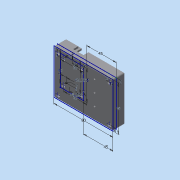
# Autodesk Inventor part: Base_V2
Saved by Autodesk Inventor 2015 (Build 190159000, 159)
## iProperties
Created: 2014-12-24
Part Number: Base_V2
Material: Generic
Document SubType Name: Modeling
Designer: Openlab
Density: 1 g/cm^3
Appearance: Default
Mass: 62.6091 g
Surface Area: 292.318 cm^2
Volume: 62.6091 cm^3
Author: Openlab
Autodesk Inventor part; units mm, degrees
ref_plane "YZ Plane" through (0, 0, 0) normal (1, 0, 0) x (0, 1, 0)
ref_plane "XZ Plane" through (0, 0, 0) normal (0, 1, 0) x (-1, 0, 0)
sketch "Sketch1" plane through (0, 0, 0) normal (0, 1, 0) x (-1, 0, 0)
  line L0 (90, 0) -> (0, 0)
  line L1 (0, 0) -> (0, -68)
  line L2 (0, -68) -> (90, -68)
  line L3 (90, -68) -> (90, 0)
  line L4 (85, -5) -> (67.5, -5)
  line L5 (5, -5) -> (5, -63)
  line L6 (5, -63) -> (85, -63)
  line L7 (85, -63) -> (85, -5)
  line L8 (35, -6.5) -> (22, -6.5)
  line L9 (22, -6.5) -> (22, -19.5)
  line L10 (22, -19.5) -> (35, -19.5)
  line L11 (35, -42.5) -> (22, -42.5)
  line L12 (22, -42.5) -> (22, -55.5)
  line L13 (22, -55.5) -> (35, -55.5)
  line L14 (85, -5) -> (81, -5)
  line L15 (81, -5) -> (81, -9)
  line L16 (81, -9) -> (85, -9)
  line L17 (85, -9) -> (85, -5)
  line L18 (85, -63) -> (81, -63)
  line L19 (81, -63) -> (81, -59)
  line L20 (81, -59) -> (85, -59)
  line L21 (85, -59) -> (85, -63)
  line L22 (5, -5) -> (9, -5)
  line L23 (9, -5) -> (9, -9)
  line L24 (9, -9) -> (5, -9)
  line L25 (5, -9) -> (5, -5)
  line L26 (5, -63) -> (9, -63)
  line L27 (9, -63) -> (9, -59)
  line L28 (9, -59) -> (5, -59)
  line L29 (5, -59) -> (5, -63)
  line L30 (67.5, -5) -> (67.5, -2.6)
  line L31 (67.5, -2.6) -> (57.5, -2.6)
  line L32 (57.5, -2.6) -> (57.5, -5)
  line L33 (67.5, -5) -> (72.2264, -5) construction
  line L34 (85, -5) -> (67.5, -5)
  line L35 (72.2264, -5) -> (57.5, -5) construction
  line L36 (57.5, -5) -> (55.2, -5)
  line L37 (12, -59) -> (12, -5)
  line L38 (40, -59) -> (12, -59)
  line L39 (12, -5) -> (5, -5)
  line L40 (36.85, -54) -> (38.15, -54)
  line L41 (38.15, -44) -> (36.85, -44)
  line L42 (35, -50.5) -> (36.85, -50.5)
  line L43 (38.15, -50.5) -> (40, -50.5)
  line L44 (40, -47.5) -> (38.15, -47.5)
  line L45 (36.85, -47.5) -> (35, -47.5)
  line L46 (36.85, -36) -> (38.15, -36)
  line L47 (38.15, -26) -> (36.85, -26)
  line L48 (40, -32.5) -> (38.15, -32.5)
  line L49 (36.85, -32.5) -> (35, -32.5)
  line L50 (40, -29.5) -> (38.15, -29.5)
  line L51 (36.85, -29.5) -> (35, -29.5)
  line L52 (35.95, -18) -> (39.05, -18)
  line L53 (39.05, -8) -> (35.95, -8)
  line L54 (35, -14.5) -> (35.95, -14.5)
  line L55 (39.05, -14.5) -> (40, -14.5)
  line L56 (35, -11.5) -> (35.95, -11.5)
  line L57 (39.05, -11.5) -> (40, -11.5)
  line L58 (12, -51.5) -> (22, -51.5)
  line L59 (12, -46.5) -> (22, -46.5)
  line L60 (12, -33.5) -> (22, -33.5)
  line L61 (12, -28.5) -> (22, -28.5)
  line L62 (12, -15.5) -> (22, -15.5)
  line L63 (12, -10.5) -> (22, -10.5)
  line L64 (42, -5) -> (42, -55)
  line L65 (57.5, -5) -> (44, -5)
  line L66 (42, -5) -> (40, -5)
  line L67 (42, -5) -> (44, -5)
  line L68 (10, -5) -> (10, -63)
  line L69 (9, -59) -> (9, -5)
  line L70 (2.6, -65.4) -> (2.6, -2.6)
  line L71 (2.6, -2.6) -> (87.4, -2.6)
  line L72 (87.4, -2.6) -> (87.4, -65.4)
  line L73 (87.4, -65.4) -> (2.6, -65.4)
  line L74 (42, -55) -> (44, -55)
  line L75 (44, -55) -> (44, -5)
  line L76 (42.1668, -13) -> (13.95, -13) construction
  line L77 (35, -6.5) -> (35, -19.5)
  line L78 (37.5, -5.5957) -> (37.5, -61.9523) construction
  line L79 (39.05, -8) -> (39.05, -18)
  line L80 (35.95, -8) -> (35.95, -18)
  line L81 (44.1467, -31) -> (11.3232, -31) construction
  line L82 (38.15, -26) -> (38.15, -36)
  line L83 (36.85, -26) -> (36.85, -36)
  line L84 (13.6727, -49) -> (43.8542, -49) construction
  line L85 (38.15, -44) -> (38.15, -54)
  line L86 (36.85, -44) -> (36.85, -54)
  line L87 (40, -5) -> (40, -59)
  line L88 (35, -42.5) -> (35, -55.5)
  line L89 (35, -24.5) -> (22, -24.5)
  line L90 (22, -24.5) -> (22, -37.5)
  line L91 (22, -37.5) -> (35, -37.5)
  line L92 (35, -37.5) -> (35, -24.5)
  line L93 (44, -63) -> (44, -61)
  line L94 (44, -61) -> (38, -61)
  line L95 (38, -61) -> (38, -63)
  line L96 (28.5, -5.8794) -> (28.5, -56.7788) construction
  point P0 (28.5, -13)
  point P1 (28.5, -31)
  point P2 (28.5, -49)
  dimension "d1" = 5
  dimension "d2" = 5
  dimension "d3" = 5
  dimension "d4" = 5
  dimension "d32" = 13
  dimension "d55" = 4
  dimension "d56" = 4
  dimension "d57" = 4
  dimension "d58" = 4
  dimension "d60" = 4
  dimension "d61" = 4
  dimension "d62" = 4
  dimension "d186" = 10
  dimension "d197" = 68
  dimension "d234" = 1.3
  dimension "d235" = 10
  dimension "d253" = 3
  dimension "d254" = 1.3
  dimension "d255" = 10
  dimension "d265" = 3
  dimension "d266" = 3.1
  dimension "d267" = 10
  dimension "d273" = 5
  dimension "d275" = 5
  dimension "d277" = 5
  dimension "d297" = 10
  dimension "d364" = 22.5
  dimension "d371" = 2.6
  dimension "d372" = 2.6
  dimension "d373" = 2.6
  dimension "d374" = 2.6
  dimension "d386" = 2
  dimension "d395" = 13
  dimension "d401" = 18
  dimension "d402" = 18
  dimension "d405" = 13
  dimension "d406" = 5
  dimension "d407" = 2
  dimension "d408" = 3
  dimension "d410" = 13
  dimension "d441" = 2
  dimension "d444" = 13
  dimension "d449" = 5
  dimension "d451" = 6.5
  dimension "d452" = 12.5
  dimension "d453" = 3.5
  dimension "d454" = 1
  dimension "d455" = 2
  dimension "d456" = 6
  dimension "d461" = 4
  dimension "d462" = 90
  dimension "d471" = 50
  constraints: 194 end point, 48 point on line, 32 perpendicular, 30 parallel, 25 horizontal, 13 collinear, 11 vertical, 1 coincident, 17 other
  measures "d1" distance between parallel lines of L2 L6
  measures "d2" distance between parallel lines of L7 L3
  measures "d3" distance between parallel lines of L1 L5
  measures "d4" distance between parallel lines of L4 L0
  measures "d32" distance of L13.end L11.start
  measures "d55" distance of L16.end L15.end
  measures "d56" distance of L15.end L14.end
  measures "d57" distance of L19.end L20.end
  measures "d58" distance of L18.end L19.end
  measures "d60" distance of L22.end L23.end
  measures "d61" distance of L28.end L27.end
  measures "d62" distance of L27.end L26.end
  measures "d186" distance of L30.end L31.end
  measures "d197" distance between parallel lines of L0 L2
  measures "d234" distance of L41.start L41.end
  measures "d235" distance of L40.end L41.start
  measures "d253" distance between parallel lines of L45 L42
  measures "d254" distance of L47.end L47.start
  measures "d255" distance of L47.start L46.end
  measures "d265" distance between parallel lines of L50 L48
  measures "d266" distance of L53.end L53.start
  measures "d267" distance of L53.start L52.end
  measures "d273" distance between parallel lines of L63 L62
  measures "d275" distance between parallel lines of L61 L60
  measures "d277" distance between parallel lines of L58 L59
  measures "d297" distance between parallel lines of L12 L37
  measures "d364" distance between parallel lines of L3 L30
  measures "d371" distance between parallel lines of L1 L70
  measures "d372" distance between parallel lines of L0 L71
  measures "d373" distance between parallel lines of L2 L73
  measures "d374" distance between parallel lines of L3 L72
  measures "d386" distance of L64.end L74.end
  measures "d395" distance between parallel lines of L10 L8
  measures "d401" distance between parallel lines of L81 L76
  measures "d402" distance between parallel lines of L84 L81
  measures "d405" distance between parallel lines of L12 L88
  measures "d406" distance between parallel lines of L88 L87
  measures "d407" distance between parallel lines of L87 L64
  measures "d408" distance between parallel lines of L54 L56
  measures "d410" distance between parallel lines of L91 L89
  measures "d441" distance between parallel lines of L68 L37
  measures "d444" distance between parallel lines of L0 L76
  measures "d449" distance between parallel lines of L0 L22
  measures "d451" distance between parallel lines of L0 L8
  measures "d452" distance between parallel lines of L2 L13
  measures "d453" distance between parallel lines of L38 L13
  measures "d454" distance between parallel lines of L27 L68
  measures "d455" distance of L93.start L93.end
  measures "d456" distance of L93.end L94.end
  measures "d461" distance of L23.end L24.end
  measures "d462" distance between parallel lines of L1 L3
  measures "d471" distance between parallel lines of L74 L65
extrude "Extrusion1" add sketch "Sketch1" against normal blind 5 contours L3 L2 L1 L0 | L7 L16 L15 L4 | L4 L30 L71 L72 L73 L70 L32 L36 L65 L67 L66 L87 L57 L79 L53 L80 L56 L77 L8 L9 L63 L37 L39 L22 L5 L6 L7 | L15 L16 L7 L20 L19 L6 L93 L94 L95 L68 L39 L37 L38 L87 L66 L64 L74 L75 L65 L36 L32 L31 L30 L4 | L7 L6 L19 L20 | L6 L95 L94 L93 | L75 L74 L64 L67 | L6 L27 L69 L23 L39 L68 | L6 L5 L28 L27 | L28 L5 L24 L69 | L23 L24 L5 L22 | L87 L55 L79 L57 | L63 L9 L62 L37 | L79 L52 L80 L53 | L87 L50 L82 L47 L83 L51 L92 L89 L90 L61 L37 L62 L9 L10 L77 L54 L80 L52 L79 L55 | L9 L8 L77 L10 | L87 L48 L82 L50 | L61 L90 L60 L37 | L82 L46 L83 L47 | L87 L44 L85 L41 L86 L45 L88 L11 L12 L59 L37 L60 L90 L91 L92 L49 L83 L46 L82 L48 | L90 L89 L92 L91 | L80 L54 L77 L56 | L87 L43 L85 L44 | L59 L12 L58 L37 | L85 L40 L86 L41 | L87 L38 L37 L58 L12 L13 L88 L42 L86 L40 L85 L43 | L12 L11 L88 L13 | L83 L49 L92 L51 | L86 L42 L88 L45
sketch "Sketch3" plane through (0, 0, 0) normal (0, 1, 0) x (-1, 0, 0)
  line L0 (45, -5) -> (45, -50)
  line L1 (80, -50) -> (80, -5)
  line L2 (80, -5) -> (45, -5)
  line L3 (45, -50) -> (80, -50)
  line L4 (71.771, -5) -> (53.229, -5)
  line L5 (53.229, -5) -> (53.229, -48.18)
  line L6 (53.229, -48.18) -> (71.771, -48.18)
  line L7 (71.771, -48.18) -> (71.771, -5)
  line L8 (62.5, 1.7089) -> (62.5, -57.768) construction
  line L9 (66.5, -10) -> (58.5, -10)
  line L10 (58.5, -10) -> (58.5, -5)
  line L11 (58.5, -5) -> (66.5, -5)
  line L12 (66.5, -5) -> (66.5, -10)
  circle A0 centre (76, -45) radius 3.5
  circle A1 centre (49, -45) radius 3.5
  circle A2 centre (76, -10) radius 3.5
  circle A3 centre (49, -10) radius 3.5
  point P0 (0, 0)
  dimension "d37" = 35
  dimension "d38" = 45
  dimension "d39" = 5
  dimension "d40" = 4
  dimension "d41" = 5
  dimension "d42" = 4
  dimension "d43" = 18.542
  dimension "d44" = 43.18
  dimension "d45" = 8
  dimension "d46" = 5
  dimension "d47" = 45
  dimension "d48" = 5
  dimension "d148" = 7
  dimension "d149" = 7
  dimension "d150" = 7
  dimension "d151" = 7
  constraints: 26 end point, 6 parallel, 5 coincident, 4 centre point, 4 horizontal alignment, 3 horizontal, 3 perpendicular, 2 vertical alignment, 1 vertical, 3 other
  measures "d37" distance of L1.start L0.end
  measures "d38" distance of L1.end L1.start
  measures "d39" distance from line of L2 point (76, -10)
  measures "d40" distance from line of L1 point (76, -45)
  measures "d41" distance from line of L3 point (76, -45)
  measures "d42" distance from line of L0 point (49, -10)
  measures "d43" distance of L5.end L6.end
  measures "d44" distance of L4.end L5.end
  measures "d45" distance of L9.start L9.end
  measures "d46" distance of L11.end L9.start
  measures "d47" distance from line of point (0, 0) L0
  measures "d48" vertical distance of point (0, 0) point (45, -5)
  measures "d148" diameter of A0
  measures "d149" diameter of A1
  measures "d150" diameter of A2
  measures "d151" diameter of A3
extrude "Extrusion4" add sketch "Sketch3" along normal blind 2 contours A0 | A1 | A2 | A3
sketch "Sketch5" plane through (0, -5, 0) normal (0, -1, 0) x (1, 0, 0)
  line L0 (-90, 0) -> (0, 0)
  line L1 (0, 0) -> (0, -68)
  line L2 (0, -68) -> (-90, -68)
  line L3 (-90, -68) -> (-90, 0)
  line L4 (-45, -5) -> (-45, -50)
  line L5 (-80, -50) -> (-80, -5)
  line L6 (-45, -50) -> (-80, -50)
  line L7 (-80, -5) -> (-45, -5)
  point P0 (-84, -62)
  point P1 (-84, -6)
  point P2 (-6, -6)
  point P3 (-6, -62)
  point P4 (-49, -10)
  point P5 (-76, -10)
  point P6 (-76, -45)
  point P7 (-49, -45)
  dimension "d310" = 90
  dimension "d311" = 68
  dimension "d314" = 6
  dimension "d315" = 6
  dimension "d316" = 6
  dimension "d317" = 6
  dimension "d326" = 45
  dimension "d342" = 35
  dimension "d347" = 4
  dimension "d352" = 4
  dimension "d353" = 5
  dimension "d354" = 5
  dimension "d355" = 45
  dimension "d356" = 5
  constraints: 16 end point, 4 horizontal alignment, 4 parallel, 4 vertical alignment, 2 coincident, 2 perpendicular, 1 horizontal
  measures "d310" distance of L1.end L2.end
  measures "d311" distance of L0.end L1.end
  measures "d314" distance from line of L0 point (-6, -6)
  measures "d315" distance from line of L1 point (-6, -6)
  measures "d316" distance from line of L2 point (-6, -62)
  measures "d317" distance from line of L3 point (-84, -6)
  measures "d326" distance of L4.end L4.start
  measures "d342" distance of L5.end L4.start
  measures "d347" distance from line of L5 point (-76, -10)
  measures "d352" distance from line of L4 point (-49, -10)
  measures "d353" distance from line of L7 point (-49, -10)
  measures "d354" distance from line of L6 point (-49, -45)
  measures "d355" distance between parallel lines of L1 L4
  measures "d356" distance between parallel lines of L0 L7
hole "Hole22" at (-49, -5, -10) at (-76, -5, -10) at (-76, -5, -45) at (-49, -5, -45) direction (0, 1, 0) diameter 4 end through all counterbore diameter 6.5 counterbore depth 3
extrude "Extrusion16" add sketch "Sketch1" along normal blind 12.5
sketch "Sketch7" plane through (-90, -5, 0) normal (0, 0, 1) x (1, 0, 0)
  line L0 (19.5, 17.5) -> (35.5, 17.5)
  line L1 (35.5, 17.5) -> (35.5, 10)
  line L2 (35.5, 10) -> (19.5, 10)
  line L3 (19.5, 10) -> (19.5, 17.5)
  line L4 (0, 17.5) -> (0, 0) projected
  point P0 (90, 5)
  dimension "d380" = 16
  dimension "d381" = 7.5
  dimension "d382" = 19.5
  dimension "d383" = 10
  constraints: 8 end point, 2 parallel, 1 horizontal, 1 perpendicular
  measures "d380" distance of L1.end L2.end
  measures "d381" distance of L0.end L1.end
  measures "d382" distance between parallel lines of L4 L3
  measures "d383" distance from line of L4.end L2
extrude "Extrusion17" cut sketch "Sketch7" against normal blind 12.5
extrude "Extrusion19" add sketch "Sketch1" along normal blind 15 contours L7 L16 L15 L4 | L4 L30 L71 L72 L73 L70 L32 L36 L65 L67 L66 L87 L57 L79 L53 L80 L56 L77 L8 L9 L63 L37 L39 L22 L5 L6 L7 | L7 L6 L19 L20 | L6 L5 L28 L27 | L23 L24 L5 L22 | L87 L50 L82 L47 L83 L51 L92 L89 L90 L61 L37 L62 L9 L10 L77 L54 L80 L52 L79 L55 | L87 L44 L85 L41 L86 L45 L88 L11 L12 L59 L37 L60 L90 L91 L92 L49 L83 L46 L82 L48 | L87 L38 L37 L58 L12 L13 L88 L42 L86 L40 L85 L43
extrude "Extrusion20" add sketch "Sketch1" along normal blind 7.4 contours L87 L55 L79 L57 | L63 L9 L62 L37 | L87 L48 L82 L50 | L61 L90 L60 L37 | L80 L54 L77 L56 | L87 L43 L85 L44 | L59 L12 L58 L37 | L83 L49 L92 L51 | L86 L42 L88 L45
extrude "Extrusion21" add sketch "Sketch1" along normal blind 2.5 contours L79 L52 L80 L53 | L82 L46 L83 L47 | L85 L40 L86 L41
hole "Hole21" at (-6, -5, -6) at (-84, -5, -6) at (-84, -5, -62) at (-6, -5, -62) direction (0, 1, 0) diameter 4 end through all counterbore diameter 6.5 counterbore depth 3
fillet "Fillet4" radius 2.5 6 edges at (-17, 7.4, -51.5) (-17, 7.4, -46.5) (-17, 7.4, -33.5) (-17, 7.4, -28.5) (-17, 7.4, -15.5) (-17, 7.4, -10.5)
sketch "Sketch9" plane through (-12, 0, -5) normal (1, 0, 0) x (0, 0, -1)
  point P0 (-5, 0)
ref_plane "Work Plane1" through (-12, 0, -5) normal (1, 0, 0) x (0, 0, -1)
sketch "Sketch10" plane through (-12, -5, 0) normal (1, 0, 0) x (0, 0, -1)
  line L0 (80, 0) -> (0, 0) construction
  arc A0 (10, 15) -> (16, 15) centre (13, 15) ccw
  arc A1 (28, 15) -> (34, 15) centre (31, 15) ccw
  arc A2 (46, 15) -> (52, 15) centre (49, 15) ccw
  line L1 (10, 15) -> (10, 20)
  line L2 (10, 20) -> (16, 20)
  line L3 (16, 20) -> (16, 15)
  line L4 (28, 15) -> (28, 20)
  line L5 (28, 20) -> (34, 20)
  line L6 (34, 20) -> (34, 15)
  line L7 (46, 15) -> (46, 20)
  line L8 (46, 20) -> (52, 20)
  line L9 (52, 20) -> (52, 15)
  line L10 (59, 5) -> (59, 20) projected
  line L11 (51.5, 20) -> (59, 20) projected
  line L12 (9, 5) -> (59, 5) projected
  line L13 (0, 0) -> (0, 17.5) projected
  point P0 (0, 5)
  point P1 (59, 7.5)
  dimension "d423" = 18
  dimension "d424" = 18
  dimension "d425" = 6
  dimension "d426" = 6
  dimension "d427" = 6
  dimension "d443" = 10
  dimension "d460" = 13
  constraints: 18 end point, 6 point on circle, 6 tangent, 5 perpendicular, 3 centre point, 3 coincident, 2 collinear, 2 horizontal alignment, 2 point on line, 2 vertical, 1 parallel
  measures "d423" distance of point (31, 15) point (13, 15)
  measures "d424" distance of point (49, 15) point (31, 15)
  measures "d425" diameter of A0
  measures "d426" diameter of A1
  measures "d427" diameter of A2
  measures "d443" distance from line of L12 A2.centre
  measures "d460" distance from line of L13 A0.centre
extrude "Extrusion23" cut sketch "Sketch10" against normal blind 1.5
fillet "Fillet5" radius 2 8 edges at (0, 3.75, 0) (-90, 3.75, 0) (-90, 3.75, -68) (0, 3.75, -68) (-45, -5, -68) (0, -5, -34) (-45, -5, 0) (-90, -5, -34)
extrude "Extrusion24" add sketch "Sketch1" along normal blind 2.5 contours L6 L95 L94 L93 | L75 L74 L64 L67 | L6 L27 L69 L23 L39 L68 | L28 L5 L24 L69
hole "Hole23" at (-28.5, 0, -13) at (-28.5, 0, -31) at (-28.5, 0, -49) direction (0, -1, 0) diameter 3 end through all countersink diameter 7 countersink angle 110
chamfer "Chamfer1" distance 1.5 angle 45 2 edges at (-41, 2.5, -61) (-42, 2.5, -30)
chamfer "Chamfer2" distance 1 angle 45 1 edges at (-10, 2.5, -34)
fillet "Fillet6" radius 1 4 edges at (-87.4, 13.75, -2.6) (-87.4, 13.75, -65.4) (-2.6, 13.75, -65.4) (-2.6, 13.75, -2.6)
body "Solid1"
